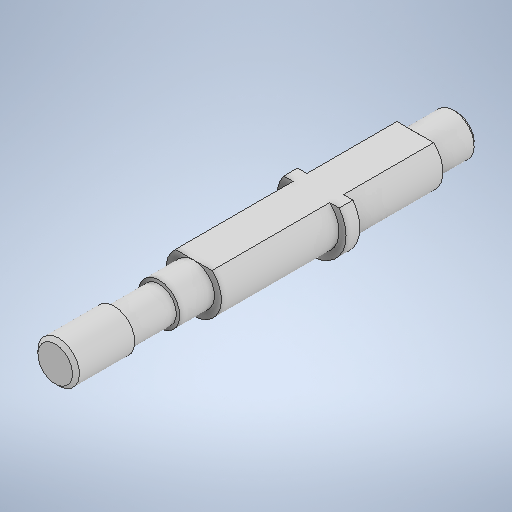
# Autodesk Inventor part: arbre_roue
Saved by Autodesk Inventor 2025.2 (Build 292293000, 293)
## iProperties
Created: 2025-03-27
Part Number: arbre_roue
Material: Générique
Document SubType Name: Modeling
Designer: enezl
Density: 1 g/cm^3
Appearance: Par défaut
Author: enezl
Autodesk Inventor part; units mm, degrees
ref_plane "YZ Plane" through (0, 0, 0) normal (1, 0, 0) x (0, 1, 0)
ref_plane "XZ Plane" through (0, 0, 0) normal (0, 1, 0) x (-1, 0, 0)
ref_plane "XY Plane" through (0, 0, 0) normal (0, 0, 1) x (1, 0, 0)
sketch "Esquisse1" plane through (0, 0, 0) normal (1, 0, 0) x (0, 1, 0)
  line L0 (0, 52) -> (3, 52)
  line L1 (3, 32) -> (4, 32)
  line L2 (4, 32) -> (4, 15)
  line L3 (4, 0) -> (3, 0)
  line L4 (3, 0) -> (3, -6)
  line L5 (3, -6) -> (0, -6)
  line L6 (0, 64.5811) -> (0, -64.5811)
  line L7 (4, 15) -> (5, 15)
  line L8 (5, 15) -> (5, 13)
  line L9 (5, 13) -> (4, 13)
  line L10 (4, 13) -> (4, 0)
  line L11 (3, 43.5) -> (2.5, 43.5)
  line L12 (2.5, 43.5) -> (2.5, 37)
  line L13 (2.5, 37) -> (3, 37)
  line L14 (3, 37) -> (3, 43.5) construction
  line L15 (3, 52) -> (3, 43.5)
  line L16 (3, 37) -> (3, 32)
  point P0 (0, 0)
  dimension "d1" = 6
  dimension "d3" = 8
  dimension "d4" = 2
  dimension "d5" = 10
  dimension "d6" = 13
  dimension "d7" = 17
  dimension "d8" = 20
  dimension "d9" = 6
  dimension "d16" = 0.5
  dimension "d17" = 8.5
  dimension "d18" = 5
  constraints: 34 end point, 13 perpendicular, 4 point on line, 3 horizontal, 2 midpoint, 2 parallel, 1 collinear, 1 vertical
  measures "d1" diameter of L4 L6
  measures "d3" diameter of L2 L6
  measures "d4" distance of L7.end L8.end
  measures "d5" diameter of L8 L6
  measures "d6" distance between parallel lines of L9 L3
  measures "d7" distance between parallel lines of L1 L7
  measures "d8" distance of L0.end L1.start
  measures "d9" distance of L3.end L4.end
  measures "d16" distance of L11.start L11.end
  measures "d17" distance between parallel lines of L0 L11
  measures "d18" distance between parallel lines of L1 L13
revolve "Révolution1" add sketch "Esquisse1" angle 360 about axis through (0, 0, 64.5811) along (0, 0, -1)
sketch "Esquisse2" plane through (0, 0, 0) normal (1, 0, 0) x (0, 1, 0)
  line L0 (7, 32) -> (3, 32)
  line L1 (3, 32) -> (3, 0)
  line L2 (3, 0) -> (7, 0)
  line L3 (7, 0) -> (7, 32)
  line L4 (-4, 0) -> (4, 0) projected
  line L5 (-4, 32) -> (4, 32) projected
  point P0 (0, 0)
  point P1 (0, 0)
  dimension "d11" = 3
  dimension "d12" = 4
  constraints: 8 end point, 2 parallel, 2 point on line, 1 horizontal, 1 midpoint, 1 perpendicular
  measures "d11" distance from line of L1 point (0, 0)
  measures "d12" distance between parallel lines of L3 L1
extrude "Extrusion1" cut sketch "Esquisse2" along normal through all both and the other way through all
chamfer "Chanfrein1" distance 0.5 angle 45 2 edges at (0, -3, 52) (0, -3, -6)
